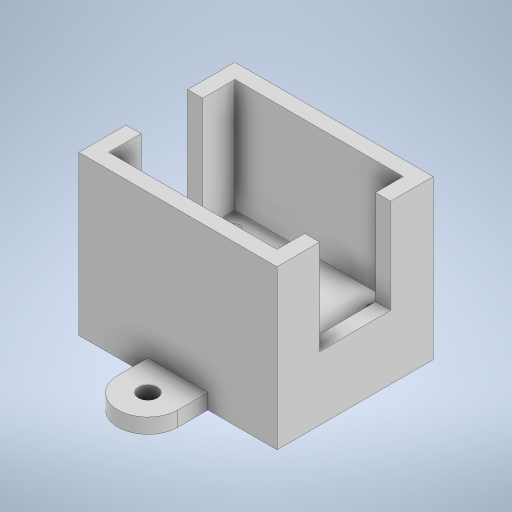
# Autodesk Inventor part: pololuCaseBottom
Saved by Autodesk Inventor 2024 (Build 280153000, 153)
## iProperties
Created: 2023-08-07
Part Number: pololuCaseBottom
Material: Generic
Document SubType Name: Modeling
Designer: 18179
Density: 1 g/cm^3
Appearance: Default
Author: 18179
Autodesk Inventor part; units mm, degrees
ref_plane "YZ Plane" through (0, 0, 0) normal (1, 0, 0) x (0, 1, 0)
ref_plane "XZ Plane" through (0, 0, 0) normal (0, 1, 0) x (-1, 0, 0)
ref_plane "XY Plane" through (0, 0, 0) normal (0, 0, 1) x (1, 0, 0)
sketch "Sketch1" plane through (0, 0, 0) normal (0, 1, 0) x (-1, 0, 0)
  line L0 (0, 0) -> (-34.29, 0)
  line L1 (-34.29, 0) -> (-34.29, 25.4)
  line L2 (-34.29, 25.4) -> (0, 25.4)
  line L3 (0, 25.4) -> (0, 0)
  line L4 (0, 25.4) -> (-2.54, 25.4) construction
  line L5 (-2.54, 25.4) -> (-2.54, 22.86) construction
  line L6 (-2.54, 22.86) -> (0, 22.86) construction
  line L7 (0, 22.86) -> (0, 25.4) construction
  line L8 (0, 0) -> (-2.54, 0) construction
  line L9 (-2.54, 0) -> (-2.54, 2.54) construction
  line L10 (-2.54, 2.54) -> (0, 2.54) construction
  line L11 (0, 2.54) -> (0, 0) construction
  line L12 (-34.29, 25.4) -> (-31.75, 25.4) construction
  line L13 (-31.75, 25.4) -> (-31.75, 22.86) construction
  line L14 (-31.75, 22.86) -> (-34.29, 22.86) construction
  line L15 (-34.29, 22.86) -> (-34.29, 25.4) construction
  line L16 (-34.29, 0) -> (-31.75, 0) construction
  line L17 (-31.75, 0) -> (-31.75, 2.54) construction
  line L18 (-31.75, 2.54) -> (-34.29, 2.54) construction
  line L19 (-34.29, 2.54) -> (-34.29, 0) construction
  circle A0 centre (-2.54, 22.86) radius 1.0922
  circle A1 centre (-2.54, 2.54) radius 1.0922
  circle A2 centre (-31.75, 2.54) radius 1.0922
  circle A3 centre (-31.75, 22.86) radius 1.0922
  line L20 (0.635, 26.035) -> (-34.925, 26.035)
  line L21 (-34.925, 26.035) -> (-34.925, -0.635)
  line L22 (-34.925, -0.635) -> (0.635, -0.635)
  line L23 (0.635, -0.635) -> (0.635, 26.035)
  dimension "d0" = 34.29
  dimension "d1" = 25.4
  dimension "d2" = 2.54
  dimension "d3" = 2.54
  dimension "d4" = 2.54
  dimension "d5" = 2.54
  dimension "d6" = 2.54
  dimension "d7" = 2.54
  dimension "d8" = 2.54
  dimension "d9" = 2.54
  dimension "d10" = 2.1844
  dimension "d11" = 2.1844
  dimension "d12" = 2.1844
  dimension "d13" = 2.1844
  dimension "d14" = 0.635
  constraints: 48 end point, 12 parallel, 6 perpendicular, 5 horizontal, 4 centre point, 4 coincident, 3 other
  measures "d0" distance of L1.end L2.end
  measures "d1" distance of L2.end L0.start
  measures "d2" distance of L6.end L5.end
  measures "d3" distance of L5.end L4.end
  measures "d4" distance of L9.end L10.end
  measures "d5" distance of L8.end L9.end
  measures "d6" distance of L13.end L14.end
  measures "d7" distance of L12.end L13.end
  measures "d8" distance of L18.end L17.end
  measures "d9" distance of L17.end L16.end
  measures "d10" diameter of A0
  measures "d11" diameter of A1
  measures "d12" diameter of A2
  measures "d13" diameter of A3
  measures "d14" distance between parallel lines of L2 L20
extrude "Extrusion1" add sketch "Sketch1" along normal blind 3.175 contours L0 L1 L2 L3 | L23 L22 L21 L20
sketch "Sketch2" plane through (0, 3.175, 0) normal (0, 1, 0) x (1, 0, 0)
  line L0 (34.925, -26.035) -> (34.925, 0.635) projected
  line L1 (34.925, 0.635) -> (-0.635, 0.635) projected
  line L2 (-0.635, 0.635) -> (-0.635, -26.035) projected
  line L3 (-0.635, -26.035) -> (34.925, -26.035) projected
  circle A0 centre (2.54, -22.86) radius 1.0922 projected
  circle A1 centre (2.54, -2.54) radius 1.0922 projected
  circle A2 centre (31.75, -2.54) radius 1.0922 projected
  circle A3 centre (31.75, -22.86) radius 1.0922 projected
  line L4 (-3.81, -29.21) -> (-3.81, 3.81)
  line L5 (-3.81, 3.81) -> (38.1, 3.81)
  line L6 (38.1, 3.81) -> (38.1, -29.21)
  line L7 (38.1, -29.21) -> (-3.81, -29.21)
  point P0 (0, 0)
  dimension "d17" = 3.175
  constraints: 8 end point, 3 other
  measures "d17" distance between parallel lines of L2 L4
extrude "Extrusion2" add sketch "Sketch2" along normal blind 24 and the other way blind 3.175 contours L4 L5 L6 L7
sketch "Sketch3" plane through (38.1, 0, -3.81) normal (1, 0, 0) x (0, 0, -1)
  line L0 (-3.175, 27.175) -> (-29.845, 27.175) projected
  line L1 (-16.51, 27.175) -> (-24.01, 27.175)
  line L2 (-24.01, 27.175) -> (-9.01, 27.175)
  line L3 (-9.01, 27.175) -> (-9.01, 3.175)
  line L4 (-29.845, 3.175) -> (-3.175, 3.175) projected
  line L5 (-24.01, 27.175) -> (-24.01, 3.175)
  point P0 (-3.81, 0)
  dimension "d22" = 7.5
  dimension "d23" = 15
  constraints: 8 end point, 3 point on line, 1 midpoint, 1 perpendicular, 1 vertical
  measures "d22" distance of L1.start L1.end
  measures "d23" distance of L1.end L2.end
extrude "Extrusion3" cut sketch "Sketch3" against normal blind 24
sketch "Sketch4" plane through (-0.635, 3.175, 26.035) normal (1, 0, 0) x (0, 0, -1)
  line L0 (29.845, 24) -> (-3.175, 24) projected
  line L1 (13.335, 24) -> (6.835, 24)
  line L2 (6.835, 24) -> (19.835, 24)
  line L3 (26.67, 0) -> (0, 0) projected
  line L4 (19.835, 24) -> (6.835, 24)
  line L5 (6.835, 24) -> (6.835, 0)
  line L6 (6.835, 0) -> (19.835, 0)
  line L7 (19.835, 0) -> (19.835, 24)
  point P0 (26.035, -3.175)
  dimension "d26" = 6.5
  dimension "d27" = 13
  constraints: 12 end point, 3 point on line, 2 parallel, 1 horizontal, 1 midpoint, 1 perpendicular
  measures "d26" distance of L1.start L1.end
  measures "d27" distance of L1.end L2.end
extrude "Extrusion4" cut sketch "Sketch4" against normal blind 24
sketch "Sketch5" plane through (0, 0, 0) normal (0, -1, 0) x (1, 0, 0)
  line L0 (38.1, -3.81) -> (38.1, 29.21) projected
  line L1 (38.1, 29.21) -> (-3.81, 29.21) projected
  line L2 (-3.81, 29.21) -> (-3.81, -3.81) projected
  line L3 (-3.81, -3.81) -> (38.1, -3.81) projected
  circle A0 centre (2.54, 22.86) radius 1.0922 projected
  circle A1 centre (2.54, 2.54) radius 1.0922 projected
  circle A2 centre (31.75, 2.54) radius 1.0922 projected
  circle A3 centre (31.75, 22.86) radius 1.0922 projected
  line L4 (-0.635, -0.635) -> (-0.635, 26.035)
  line L5 (-0.635, 26.035) -> (34.925, 26.035)
  line L6 (34.925, 26.035) -> (34.925, -0.635)
  line L7 (34.925, -0.635) -> (-0.635, -0.635)
  line L8 (17.145, 29.21) -> (17.145, 35.56)
  line L9 (17.145, -3.81) -> (17.145, -10.16)
  circle A4 centre (17.145, 35.56) radius 2
  circle A5 centre (17.145, -10.16) radius 2
  circle A6 centre (17.145, 35.56) radius 6.35
  circle A7 centre (17.145, -10.16) radius 6.35
  line L10 (23.495, 35.56) -> (23.495, 29.21)
  line L11 (10.795, 35.56) -> (10.795, 29.21)
  line L12 (10.795, -10.16) -> (10.795, -3.81)
  line L13 (23.495, -10.16) -> (23.495, -3.81)
  point P0 (0, 0)
  dimension "d30" = 3.175
  dimension "d31" = 6.35
  dimension "d32" = 6.35
  dimension "d33" = 4
  dimension "d34" = 4
  constraints: 20 end point, 6 point on circle, 4 centre point, 4 coincident, 4 perpendicular, 4 point on line, 3 tangent, 2 midpoint, 2 vertical, 3 other
  measures "d30" distance between parallel lines of L2 L4
  measures "d31" distance of L8.start L8.end
  measures "d32" distance of L9.start L9.end
  measures "d33" diameter of A4
  measures "d34" diameter of A5
extrude "Extrusion5" add sketch "Sketch5" along normal blind 6.35 contours L3 L2 L1 L0 | L13 A7 L3 | L1 A6 L10 | A7 L12 L3 | A7 | L1 L11 A6 | A6
sketch "Sketch6" plane through (0, 3.175, 0) normal (0, 1, 0) x (1, 0, 0)
  circle A0 centre (31.75, -22.86) radius 1.0922 projected
  circle A1 centre (31.75, -2.54) radius 1.0922 projected
  circle A2 centre (2.54, -2.54) radius 1.0922 projected
  circle A3 centre (2.54, -22.86) radius 1.0922 projected
  line L0 (34.925, -5.2) -> (34.925, 0.635) projected
  line L1 (34.925, 0.635) -> (-0.635, 0.635) projected
  line L2 (-0.635, 0.635) -> (-0.635, -6.2) projected
  line L3 (-0.635, -6.2) -> (-3.81, -6.2) projected
  line L4 (-3.81, -19.2) -> (-3.81, -6.2) projected
  line L5 (-0.635, -19.2) -> (-3.81, -19.2) projected
  line L6 (-0.635, -19.2) -> (-0.635, -26.035) projected
  line L7 (-0.635, -26.035) -> (34.925, -26.035) projected
  line L8 (34.925, -26.035) -> (34.925, -20.2) projected
  line L9 (38.1, -20.2) -> (34.925, -20.2) projected
  line L10 (38.1, -5.2) -> (38.1, -20.2) projected
  line L11 (38.1, -5.2) -> (34.925, -5.2) projected
  line L12 (-0.635, -6.2) -> (-0.635, -19.2)
  line L13 (34.925, -5.2) -> (34.925, -20.2)
  point P0 (0, 0)
  constraints: 4 end point, 1 parallel, 1 vertical
extrude "Extrusion6" add sketch "Sketch6" along normal blind 4 contours L11 L10 L9 L13 | L12 L5 L4 L3
sketch "Sketch7" plane through (0, 0, 0) normal (0, 1, 0) x (1, 0, 0)
  line L0 (10.795, 3.81) -> (23.495, 3.81) projected
  line L1 (23.495, 10.16) -> (23.495, 3.81) projected
  arc A0 (23.495, 10.16) -> (10.795, 10.16) centre (17.145, 10.16) ccw projected
  line L2 (10.795, 3.81) -> (10.795, 10.16) projected
  circle A1 centre (17.145, 10.16) radius 2 projected
  circle A2 centre (17.145, -35.56) radius 2 projected
  line L3 (23.495, -29.21) -> (10.795, -29.21) projected
  line L4 (10.795, -35.56) -> (10.795, -29.21) projected
  arc A3 (10.795, -35.56) -> (23.495, -35.56) centre (17.145, -35.56) ccw projected
  line L5 (23.495, -29.21) -> (23.495, -35.56) projected
  point P0 (0, 0)
extrude "Extrusion7" cut sketch "Sketch7" against normal blind 3.175
body "Solid1"
